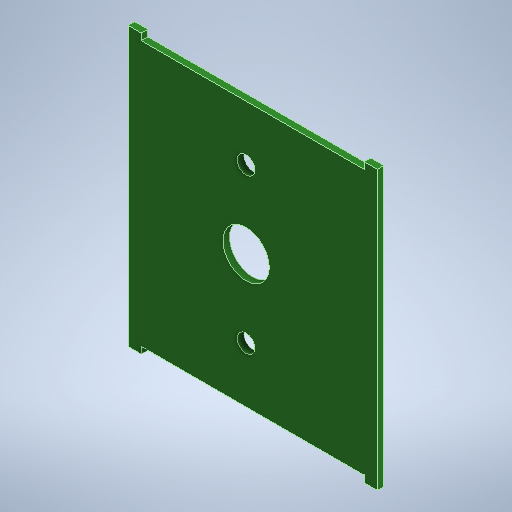
# Autodesk Inventor part: upper support
Saved by Autodesk Inventor 2025.4 (Build 294407000, 407)
## iProperties
Created: 2026-05-23
Part Number: upper support
Material: Generic
Document SubType Name: Modeling
Designer: lenovo
Density: 1 g/cm^3
Appearance: Default(1)
Author: lenovo
Autodesk Inventor part; units mm, degrees
ref_plane "YZ Plane" through (0, 0, 0) normal (1, 0, 0) x (0, 1, 0)
ref_plane "XZ Plane" through (0, 0, 0) normal (0, 1, 0) x (-1, 0, 0)
ref_plane "XY Plane" through (0, 0, 0) normal (0, 0, 1) x (1, 0, 0)
sketch "Sketch1" plane through (0, 0, 0) normal (0, 0, 1) x (1, 0, 0)
  line L0 (-56.5, -63) -> (56.5, -63)
  line L1 (56.5, -63) -> (56.5, 63)
  line L2 (56.5, 63) -> (-56.5, 63)
  line L3 (-56.5, 63) -> (-56.5, -63)
  line L4 (-56.5, -63) -> (56.5, 63) construction
  line L5 (56.5, -63) -> (-56.5, 63) construction
  line L6 (56.5, -63) -> (50.5, -63)
  line L7 (50.5, -63) -> (50.5, -60)
  line L8 (50.5, -60) -> (56.5, -60)
  line L9 (56.5, -60) -> (56.5, -63)
  line L10 (0, 63) -> (0, -63)
  line L11 (-56.5, 0) -> (56.5, 0)
  line L12 (-56.5, -63) -> (-50.5, -63)
  line L13 (-50.5, -63) -> (-50.5, -60)
  line L14 (-50.5, -60) -> (-56.5, -60)
  line L15 (-56.5, -60) -> (-56.5, -63)
  line L16 (50.5, 63) -> (50.5, 60)
  line L17 (50.5, 60) -> (56.5, 60)
  line L18 (-50.5, 63) -> (-50.5, 60)
  line L19 (-50.5, 60) -> (-56.5, 60)
  line L20 (-50.5, -60) -> (50.5, -60)
  line L21 (-50.5, 60) -> (50.5, 60)
  point P0 (0, 0)
  point P1 (-50.5, -63)
  point P2 (50.5, -63)
  point P3 (50.5, 63)
  point P4 (-50.5, 63)
  dimension "d0" = 113
  dimension "d1" = 126
  dimension "d2" = 6
  dimension "d3" = 3
  constraints: 44 end point, 9 symmetric about line, 6 midpoint, 6 parallel, 2 horizontal, 2 perpendicular
  measures "d0" distance of L1.end L2.end
  measures "d1" distance of L0.end L1.end
  measures "d2" distance of L7.end L8.end
  measures "d3" distance of L6.end L7.end
extrude "Extrusion1" add sketch "Sketch1" along normal mid plane 3 contours L3 L14 L13 L0 | L3 L11 L10 L20 L14 | L3 L19 L21 L10 L11 | L7 L8 L1 L0 | L10 L11 L1 L8 L20 | L3 L2 L18 L19 | L10 L21 L17 L1 L11 | L16 L2 L1 L17
sketch "Sketch2" plane through (0, 0, 1.5) normal (0, 0, 1) x (1, 0, 0)
  circle A0 centre (-3, -35) radius 4
  line L0 (-3, 0) -> (-56.5, 0)
  line L1 (-56.5, 63) -> (-56.5, -63) projected
  circle A1 centre (-3, 35) radius 4
  circle A2 centre (-3, 0) radius 10.5
  line L2 (56.5, -63) -> (56.5, 63) projected
  line L3 (50.5, 60) -> (-50.5, 60) projected
  dimension "d6" = 70
  dimension "d7" = 8
  dimension "d8" = 21
  dimension "d11" = 59.5
  dimension "d12" = 60
  constraints: 3 centre point, 3 vertical alignment, 2 end point, 1 horizontal, 1 midpoint, 1 symmetric about line, 1 other
  measures "d6" diameter of A0.centre L0
  measures "d7" diameter of A0
  measures "d8" diameter of A2
  measures "d11" distance from line of L2 A2.centre
  measures "d12" distance from line of L3 A2.centre
extrude "Extrusion2" cut sketch "Sketch2" against normal blind 3
body "Solid1"
